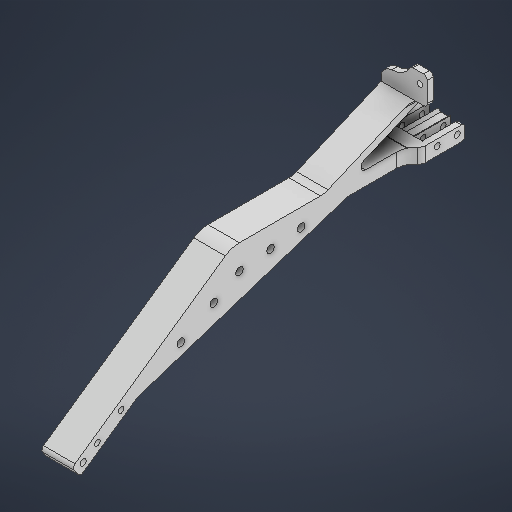
# Autodesk Inventor part: палка
Saved by Autodesk Inventor 2025 (Build 290162000, 162)
## iProperties
Created: 2025-01-21
Part Number: палка
Material: Типовые
Document SubType Name: Modeling
Designer: Phantom
Density: 1 g/cm^3
Appearance: По умолчанию
Author: Phantom
Autodesk Inventor part; units mm, degrees
ref_plane "YZ Plane" through (0, 0, 0) normal (1, 0, 0) x (0, 1, 0)
ref_plane "XZ Plane" through (0, 0, 0) normal (0, 1, 0) x (-1, 0, 0)
ref_plane "XY Plane" through (0, 0, 0) normal (0, 0, 1) x (1, 0, 0)
sketch "Эскиз1" plane through (0, 0, 0) normal (0, 0, 1) x (1, 0, 0)
  line L0 (6.1329, 20.7465) -> (8.1329, 22.2465)
  line L1 (8.1329, 22.2465) -> (8.1329, 14.2465)
  line L2 (8.1329, 14.2465) -> (6.1329, 15.7465)
  line L3 (6.1329, 15.7465) -> (2.1329, 15.7465)
  line L4 (2.1329, 15.7465) -> (0.1329, 14.2465)
  line L5 (0.1329, 14.2465) -> (0.1329, 22.2465)
  line L6 (0.1329, 22.2465) -> (2.1329, 20.7465)
  line L7 (6.1329, 20.7465) -> (2.1329, 20.7465)
  point P0 (0, 0)
  constraints: 16 end point
extrude "Выдавливание1" add sketch "Эскиз1" along normal blind 20
sketch "Эскиз2" plane through (8.1329, 14.2465, 0) normal (1, 0, 0) x (0, 0, -1)
  line L0 (-20, 0) -> (-20, 1.5) projected
  line L1 (-20, 6.5) -> (-20, 8) projected
  line L2 (-20, 8) -> (-20, 0)
  line L3 (-172, -60) -> (-160, -60) construction
  line L4 (-172, -37) -> (-205, -60)
  line L5 (-172, -37) -> (-20, 0)
  line L6 (-20, 8) -> (-175.1358, -29.7633)
  line L7 (-209.42, -53.6583) -> (-175.1358, -29.7633)
  line L8 (-205, -60) -> (-209.42, -53.6583)
  point P0 (0, -14.2465)
  constraints: 14 end point, 2 parallel, 1 horizontal, 1 perpendicular, 1 other
extrude "Выдавливание2" add sketch "Эскиз2" against normal up to surface (8 mm away)
sketch "Эскиз3" plane through (8.1329, 22.2465, 20) normal (0, 0, -1) x (-1, 0, 0)
  line L0 (0, 0) -> (2, -1.5) projected
  line L1 (2, -1.5) -> (6, -1.5) projected
  line L2 (6, -1.5) -> (8, 0) projected
  line L3 (0, 0) -> (8, 0) projected
  point P0 (8.1329, -22.2465)
extrude "Выдавливание3" cut sketch "Эскиз3" against normal blind 10
sketch "Эскиз4" plane through (0, 0, 0) normal (0, 0, -1) x (-1, 0, 0)
  line L0 (-2.1329, 20.7465) -> (-0.1329, 22.2465) projected
  line L1 (-6.1329, 20.7465) -> (-2.1329, 20.7465) projected
  line L2 (-8.1329, 22.2465) -> (-6.1329, 20.7465) projected
  line L3 (-8.1329, 14.2465) -> (-8.1329, 22.2465) projected
  line L4 (-6.1329, 15.7465) -> (-8.1329, 14.2465) projected
  line L5 (-2.1329, 15.7465) -> (-6.1329, 15.7465) projected
  line L6 (-0.1329, 14.2465) -> (-2.1329, 15.7465) projected
  line L7 (-0.1329, 22.2465) -> (-0.1329, 14.2465) projected
  line L8 (-8.1329, 18.2465) -> (-8.1329, 14.7465)
  line L9 (-8.1329, 14.2465) -> (-8.1329, 22.2465) projected
  line L10 (-8.1329, 18.2465) -> (-8.1329, 21.7465)
  line L11 (-7.6329, 21.3715) -> (-6.1329, 20.2465)
  line L12 (-8.1329, 22.2465) -> (-6.1329, 20.7465) projected
  line L13 (-6.1329, 20.2465) -> (-2.1329, 20.2465)
  line L14 (-2.1329, 20.2465) -> (-0.6329, 21.3715)
  line L15 (-8.1329, 18.2465) -> (0, 18.2465)
  line L16 (-7.6329, 15.1215) -> (-6.1329, 16.2465)
  line L17 (-6.1329, 16.2465) -> (-2.1329, 16.2465)
  line L18 (-2.1329, 16.2465) -> (-0.6329, 15.1215)
  line L19 (-8.1329, 18.2465) -> (-7.6329, 18.2465)
  line L20 (-7.6329, 21.3715) -> (-7.6329, 15.1215)
  line L21 (-4.1329, 16.2465) -> (-4.1329, 20.2465)
  line L22 (-0.6329, 21.3715) -> (-0.6329, 15.1215)
  point P0 (0, 0)
  point P1 (-0.1329, 21.7465)
  point P2 (-0.1329, 14.7465)
  dimension "d15" = 3.5
  dimension "d16" = 3.5
  constraints: 26 end point, 5 symmetric about line, 4 midpoint, 4 point on line, 3 parallel, 1 horizontal, 1 perpendicular
  measures "d15" distance of L8.start L8.end
  measures "d16" distance of L8.start L10.end
extrude "Выдавливание4" cut sketch "Эскиз4" against normal up to surface (20 mm away) contours L0 L7 L15 L22 L14 L13 L11 L20 L3 L2 L1 | L7 L6 L5 L4 L3 L15 L20 L16 L17 L18 L22
sketch "Эскиз5" plane through (8.1329, 14.2465, 20) normal (0, 0, -1) x (-1, 0, 0)
  line L0 (-11, -14.2465) -> (13, -14.2465)
  line L1 (13, -14.2465) -> (13, 14)
  line L2 (13, 14) -> (-11, 14)
  line L3 (-11, 14) -> (-11, -14.2465)
  line L4 (0, 0) -> (8, 0) projected
  line L5 (8, 8) -> (8, 0) projected
  line L6 (6, 6.5) -> (8, 8) projected
  line L7 (2, 6.5) -> (6, 6.5) projected
  line L8 (0, 8) -> (2, 6.5) projected
  line L9 (0, 0) -> (0, 8) projected
  line L10 (2, 6) -> (0.5, 7.125) projected
  line L11 (6, 6) -> (2, 6) projected
  line L12 (7.5, 7.125) -> (6, 6) projected
  line L13 (7.5, 0.875) -> (7.5, 7.125) projected
  line L14 (6, 2) -> (7.5, 0.875) projected
  line L15 (2, 2) -> (6, 2) projected
  line L16 (0.5, 0.875) -> (2, 2) projected
  line L17 (0.5, 7.125) -> (0.5, 0.875) projected
  line L18 (0, 0.875) -> (8, 0.875)
  point P0 (8.1329, -14.2465)
  constraints: 10 end point, 2 parallel, 2 perpendicular, 2 point on line, 1 horizontal
extrude "Выдавливание5" cut sketch "Эскиз5" against normal through all contours L9 L8 L7 L6 L5 L18 L13 L12 L11 L10 L17
sketch "Эскиз8" plane through (0.1329, -15.5168, 175.1358) normal (0, 0.9716279, 0.2365147) x (1, 0, 0)
  line L0 (8, 129.5409) -> (7.5, 129.5409) projected
  line L1 (8, 157.9807) -> (8, 129.5409) projected
  line L2 (7.5, 157.9807) -> (8, 157.9807) projected
  line L3 (7.5, 157.9807) -> (7.5, 129.5409) projected
  line L4 (0.5, 129.5409) -> (0, 129.5409) projected
  line L5 (0.5, 157.9807) -> (0.5, 129.5409) projected
  line L6 (0, 157.9807) -> (0.5, 157.9807) projected
  line L7 (0, 129.5409) -> (0, 157.9807) projected
  line L8 (7.5, 129.5409) -> (61, 129.5409)
  line L9 (61, 129.5409) -> (61, -147)
  line L10 (61, -147) -> (7.5, -147)
  line L11 (7.5, -147) -> (7.5, 129.5409)
  line L12 (0.5, 129.5409) -> (-35, 129.5409)
  line L13 (-35, 129.5409) -> (-35, -116)
  line L14 (-35, -116) -> (0.5, -116)
  line L15 (0.5, -116) -> (0.5, 129.5409)
  point P0 (-0.1329, 173.8368)
  point P1 (0, 129.5409)
  point P2 (8, 129.5409)
  constraints: 16 end point, 4 parallel, 2 horizontal, 2 perpendicular
extrude "Выдавливание7" cut sketch "Эскиз8" against normal blind 10
chamfer "Фаска1" distance 2 angle 45 1 edges at (4.1329, 14.2465, 20)
sketch "Эскиз9" plane through (0.1329, -39.4118, 209.42) normal (0, 0.8203982, 0.5717927) x (1, 0, 0)
  line L0 (0, 14.1297) -> (0, 34.0646) projected
  line L1 (0, 34.0646) -> (0.5, 34.0646) projected
  line L2 (0, 14.1297) -> (0, 34.0646) projected
  line L3 (0.5, 14.1297) -> (0, 14.1297) projected
  line L4 (0.5, 34.0646) -> (0.5, 14.1297) projected
  line L5 (8, 14.1297) -> (7.5, 14.1297) projected
  line L6 (8, 34.0646) -> (8, 14.1297) projected
  line L7 (7.5, 34.0646) -> (8, 34.0646) projected
  line L8 (7.5, 14.1297) -> (7.5, 34.0646) projected
  line L9 (0.5, 14.1297) -> (-8, 14.1297)
  line L10 (-8, 14.1297) -> (-8, -12)
  line L11 (-8, -12) -> (0.5, -12)
  line L12 (0.5, -12) -> (0.5, 14.1297)
  line L13 (7.5, 14.1297) -> (11, 14.1297)
  line L14 (11, 14.1297) -> (11, -15)
  line L15 (11, -15) -> (7.5, -15)
  line L16 (7.5, -15) -> (7.5, 14.1297)
  point P0 (-0.1329, 194.3431)
  point P1 (0, 34.0646)
  constraints: 16 end point, 4 parallel, 2 horizontal, 2 perpendicular
extrude "Выдавливание8" cut sketch "Эскиз9" against normal through all
sketch "Эскиз10" plane through (0.6329, 15.1215, 0) normal (-1, 0, 0) x (0, 0, 1)
  circle A0 centre (15.2, 3.125) radius 1.6
  circle A1 centre (4.2, 3.125) radius 1.6
  line L0 (0, 6.25) -> (0, 0) projected
  line L1 (15.2, 3.125) -> (0, 3.125)
  point P0 (0, -15.1215)
  constraints: 2 centre point, 2 end point, 1 midpoint
extrude "Выдавливание9" cut sketch "Эскиз10" against normal through all
sketch "Эскиз11" plane through (0.6329, 15.1215, 0) normal (-1, 0, 0) x (0, 0, 1)
  circle A0 centre (182.5992, -40.5488) radius 1.575
  arc A1 (197.0381, -49.974) -> (196.4376, -50.8354) centre (195.5197, -49.5556) ccw
  arc A2 (204.9267, -55.4731) -> (201.6465, -55.5591) centre (203.272, -54.9596) ccw
  arc A3 (201.6174, -54.4462) -> (204.8975, -54.3601) centre (203.272, -54.9596) ccw
  line L0 (209.42, -54.5333) -> (205, -60.875) projected
  circle A4 centre (195.5197, -49.5556) radius 1.575
  point P0 (0, -15.1215)
  point P1 (203.272, -54.9596)
  point P2 (203.272, -54.9596)
  point P3 (201.6465, -55.5591)
  point P4 (204.9267, -55.4731)
  dimension "d67" = 3.15
  dimension "d68" = 1.575
  constraints: 6 point on circle, 5 centre point, 1 coincident, 1 concentric
  measures "d67" diameter of A0
  measures "d68" radius of A1
extrude "Выдавливание10" cut sketch "Эскиз11" against normal through all
fillet "Сопряжение2" radius 2 2 edges at (4.1329, -45.7535, 205) (4.1329, -39.4118, 209.42)
sketch "Эскиз12" plane through (7.6329, 15.1215, 0) normal (1, 0, 0) x (0, 0, -1)
  circle A0 centre (-195.5197, -49.5556) radius 1.575 projected
  circle A1 centre (-182.5992, -40.5488) radius 1.575 projected
  circle A2 centre (-203.272, -54.9596) radius 1.7325 projected
  circle A3 centre (-4.2, 3.125) radius 1.6 projected
  circle A4 centre (-15.2, 3.125) radius 1.6 projected
  arc A5 (-207.7792, -53.3897) -> (-208.2764, -56.1741) centre (-206.6356, -55.0305) ccw projected
  line L0 (-206.1436, -59.2342) -> (-208.2764, -56.1741) projected
  arc A6 (-206.1436, -59.2342) -> (-203.3592, -59.7314) centre (-204.5028, -58.0906) ccw projected
  line L1 (-172, -37.875) -> (-203.3592, -59.7314) projected
  line L2 (-21.9433, -1.348) -> (-172, -37.875) projected
  line L3 (-20.884, 0) -> (-21.9433, -1.348) projected
  line L4 (0, 0) -> (-20.884, 0) projected
  line L5 (0, 6.25) -> (0, 0) projected
  line L6 (0, 6.25) -> (-23.5946, 6.25) projected
  line L7 (-175.1358, -30.6383) -> (-23.5946, 6.25) projected
  line L8 (-207.7792, -53.3897) -> (-175.1358, -30.6383) projected
  line L9 (-175.1358, -30.6383) -> (-122.2091, 6.25)
  line L10 (-207.7792, -53.3897) -> (-175.1358, -30.6383) projected
  line L11 (-172, -37.875) -> (-117.6576, 0)
  line L12 (-23.5946, 6.25) -> (-122.2091, 6.25)
  line L13 (-20.884, 0) -> (-117.6576, 0)
  point P0 (0, -15.1215)
  point P1 (-154.3613, -25.5814)
  point P2 (-49.2703, 0)
  constraints: 8 end point, 1 collinear, 1 horizontal, 1 parallel
extrude "Выдавливание11" add sketch "Эскиз12" against normal up to surface (7 mm away) contours L9 L12 L7 L13 L11
sketch "Эскиз13" plane through (7.6329, 15.1215, 0) normal (1, 0, 0) x (0, 0, -1)
  line L0 (-122.2091, 6.25) -> (-207.7792, -53.3897) projected
  arc A0 (-207.7792, -53.3897) -> (-208.2764, -56.1741) centre (-206.6356, -55.0305) ccw projected
  line L1 (-206.1436, -59.2342) -> (-208.2764, -56.1741) projected
  arc A1 (-206.1436, -59.2342) -> (-203.3592, -59.7314) centre (-204.5028, -58.0906) ccw projected
  line L2 (-172, -37.875) -> (-203.3592, -59.7314) projected
  line L3 (-21.9433, -1.348) -> (-172, -37.875) projected
  line L4 (-20.884, 0) -> (-21.9433, -1.348) projected
  line L5 (0, 0) -> (-20.884, 0) projected
  line L6 (0, 6.25) -> (0, 0) projected
  line L7 (0, 6.25) -> (-23.5946, 6.25) projected
  line L8 (-23.5946, 6.25) -> (-122.2091, 6.25) projected
  circle A2 centre (-195.5197, -49.5556) radius 1.575 projected
  circle A3 centre (-182.5992, -40.5488) radius 1.575 projected
  circle A4 centre (-203.272, -54.9596) radius 1.7325 projected
  circle A5 centre (-4.2, 3.125) radius 1.6 projected
  circle A6 centre (-15.2, 3.125) radius 1.6 projected
  line L9 (-154.3613, -25.5814) -> (-117.6576, 0) projected
  line L10 (-117.6576, 0) -> (-49.2703, 0) projected
  line L11 (-154.3613, -25.5814) -> (-49.2703, 0) projected
  line L12 (-154.3613, -25.5814) -> (-172, -37.875)
  line L13 (-49.2703, 0) -> (-20.884, 0)
  point P0 (0, -15.1215)
  constraints: 4 end point, 1 collinear
extrude "Выдавливание12" cut sketch "Эскиз13" against normal blind 10 contours L4 L3 L12 L11 L13
fillet "Сопряжение3" radius 13.5 2 edges at (4.1329, 21.3715, 122.2091) (4.1329, 15.1215, 117.6576)
sketch "Эскиз14" plane through (7.6329, 15.1215, 0) normal (1, 0, 0) x (0, 0, -1)
  line L0 (-203.3592, -59.7314) -> (-121.1364, -2.4246) projected
  line L1 (-187.7019, -39.3965) -> (-48.0259, 6.25)
  line L2 (-20.884, 0) -> (-113.4172, 0) projected
  line L3 (-173.6161, -39.0014) -> (-48.7504, 1.8051)
  circle A0 centre (-195.5197, -49.5556) radius 1.575 projected
  circle A1 centre (-182.5992, -40.5488) radius 1.575 projected
  circle A2 centre (-203.272, -54.9596) radius 1.7325 projected
  circle A3 centre (-4.2, 3.125) radius 1.6 projected
  circle A4 centre (-15.2, 3.125) radius 1.6 projected
  arc A5 (-117.9687, 6.25) -> (-125.6879, 3.8254) centre (-117.9687, -7.25) ccw projected
  line L4 (-125.6879, 3.8254) -> (-207.7792, -53.3897) projected
  arc A6 (-207.7792, -53.3897) -> (-208.2764, -56.1741) centre (-206.6356, -55.0305) ccw projected
  line L5 (-206.1436, -59.2342) -> (-208.2764, -56.1741) projected
  arc A7 (-206.1436, -59.2342) -> (-203.3592, -59.7314) centre (-204.5028, -58.0906) ccw projected
  line L6 (-121.1364, -2.4246) -> (-203.3592, -59.7314) projected
  arc A8 (-113.4172, 0) -> (-121.1364, -2.4246) centre (-113.4172, -13.5) ccw projected
  line L7 (-113.4172, 0) -> (-20.884, 0) projected
  line L8 (0, 0) -> (-20.884, 0) projected
  line L9 (0, 6.25) -> (0, 0) projected
  line L10 (0, 6.25) -> (-23.5946, 6.25) projected
  line L11 (-23.5946, 6.25) -> (-117.9687, 6.25) projected
  point P0 (0, -15.1215)
  point P1 (-54.2738, 0)
  point P2 (-67.1506, 0)
  point P3 (-162.2478, -31.078)
  dimension "d43" = 4
  constraints: 4 end point, 3 point on line, 1 parallel
  measures "d43" distance between parallel lines of L1 L3
extrude "Выдавливание13" add sketch "Эскиз14" against normal up to surface (7 mm away) contours L0 L1 L2 L3
sketch "Эскиз15" plane through (7.6329, 15.1215, 0) normal (1, 0, 0) x (0, 0, -1)
  line L0 (-154, -1.48) -> (-33, -1.48)
  line L1 (-113.4172, 0) -> (-67.1506, 0) projected
  line L2 (-23.5946, 6.25) -> (-117.9687, 6.25) projected
  line L3 (-33, -1.48) -> (-20.884, -1.48)
  line L4 (-20.884, -1.48) -> (-23.5946, 6.25)
  line L5 (-54.2738, 0) -> (-20.884, 0) projected
  line L6 (0, 0) -> (-20.884, 0) projected
  line L7 (0, 6.25) -> (0, 0) projected
  line L8 (0, 6.25) -> (-23.5946, 6.25) projected
  line L9 (-23.5946, 6.25) -> (-117.9687, 6.25) projected
  arc A0 (-117.9687, 6.25) -> (-125.6879, 3.8254) centre (-117.9687, -7.25) ccw projected
  line L10 (-125.6879, 3.8254) -> (-207.7792, -53.3897) projected
  arc A1 (-207.7792, -53.3897) -> (-208.2764, -56.1741) centre (-206.6356, -55.0305) ccw projected
  line L11 (-206.1436, -59.2342) -> (-208.2764, -56.1741) projected
  arc A2 (-206.1436, -59.2342) -> (-203.3592, -59.7314) centre (-204.5028, -58.0906) ccw projected
  line L12 (-173.6161, -39.0014) -> (-203.3592, -59.7314) projected
  line L13 (-173.6161, -39.0014) -> (-54.2738, 0) projected
  circle A3 centre (-195.5197, -49.5556) radius 1.575 projected
  circle A4 centre (-182.5992, -40.5488) radius 1.575 projected
  circle A5 centre (-203.272, -54.9596) radius 1.7325 projected
  circle A6 centre (-4.2, 3.125) radius 1.6 projected
  circle A7 centre (-15.2, 3.125) radius 1.6 projected
  line L14 (-67.1506, 0) -> (-162.2478, -31.078) projected
  line L15 (-121.1364, -2.4246) -> (-162.2478, -31.078) projected
  arc A8 (-113.4172, 0) -> (-121.1364, -2.4246) centre (-113.4172, -13.5) ccw projected
  line L16 (-113.4172, 0) -> (-67.1506, 0) projected
  point P0 (0, -15.1215)
  point P1 (-21.403, 0)
  point P2 (-58.8025, -1.48)
  point P3 (-119.5629, -1.48)
  point P4 (-71.6793, -1.48)
  constraints: 6 end point, 1 horizontal, 1 parallel
extrude "Выдавливание14" add sketch "Эскиз15" against normal up to surface (7 mm away) contours A8 L1 L14 L0 | L13 L5 L4 L3 L0
fillet "Сопряжение4" radius 13.5 1 edges at (4.1329, 13.6415, 20.884)
fillet "Сопряжение5" radius 2 4 edges at (4.1329, 13.6415, 58.8025) (4.1329, -23.8799, 173.6161) (4.1329, 13.6415, 71.6793) (4.1329, -15.9565, 162.2478)
sketch "Эскиз16" plane through (7.6329, 15.1215, 0) normal (1, 0, 0) x (0, 0, -1)
  arc A0 (-27.5487, -1.48) -> (-21.403, 0) centre (-27.5487, 12.02) ccw projected
  line L0 (-21.403, 0) -> (-20.884, 0) projected
  line L1 (0, 0) -> (-20.884, 0) projected
  line L2 (0, 6.25) -> (0, 0) projected
  line L3 (0, 6.25) -> (-23.5946, 6.25) projected
  line L4 (-23.5946, 6.25) -> (-117.9687, 6.25) projected
  arc A1 (-117.9687, 6.25) -> (-125.6879, 3.8254) centre (-117.9687, -7.25) ccw projected
  line L5 (-125.6879, 3.8254) -> (-207.7792, -53.3897) projected
  arc A2 (-207.7792, -53.3897) -> (-208.2764, -56.1741) centre (-206.6356, -55.0305) ccw projected
  line L6 (-206.1436, -59.2342) -> (-208.2764, -56.1741) projected
  arc A3 (-206.1436, -59.2342) -> (-203.3592, -59.7314) centre (-204.5028, -58.0906) ccw projected
  line L7 (-173.8581, -39.17) -> (-203.3592, -59.7314) projected
  arc A4 (-173.3358, -38.9098) -> (-173.8581, -39.17) centre (-172.7145, -40.8108) ccw projected
  line L8 (-173.3358, -38.9098) -> (-59.1053, -1.5789) projected
  arc A5 (-58.484, -1.48) -> (-59.1053, -1.5789) centre (-58.484, -3.48) ccw projected
  line L9 (-58.484, -1.48) -> (-27.5487, -1.48) projected
  circle A6 centre (-195.5197, -49.5556) radius 1.575 projected
  circle A7 centre (-182.5992, -40.5488) radius 1.575 projected
  circle A8 centre (-203.272, -54.9596) radius 1.7325 projected
  circle A9 centre (-4.2, 3.125) radius 1.6 projected
  circle A10 centre (-15.2, 3.125) radius 1.6 projected
  line L10 (-83.6164, -5.3811) -> (-149.3566, -26.8651) projected
  arc A11 (-151.1214, -23.3233) -> (-149.3566, -26.8651) centre (-149.9779, -24.9641) ccw projected
  line L11 (-121.1364, -2.4246) -> (-151.1214, -23.3233) projected
  arc A12 (-119.5629, -1.48) -> (-121.1364, -2.4246) centre (-113.4172, -13.5) ccw projected
  line L12 (-119.5629, -1.48) -> (-84.2377, -1.48) projected
  arc A13 (-83.6164, -5.3811) -> (-84.2377, -1.48) centre (-84.2377, -3.48) ccw projected
  line L13 (-20.884, 0) -> (-20.884, 6.25)
  point P0 (0, -15.1215)
  constraints: 2 end point, 1 perpendicular, 1 point on line
extrude "Выдавливание15" add sketch "Эскиз16" along normal blind 2.5 contours L9 A5 L8 A4 L7 A3 L6 A2 L5 A1 L4 L3 L13 L0 A0
sketch "Эскиз17" plane through (0.6329, 15.1215, 0) normal (-1, 0, 0) x (0, 0, 1)
  circle A0 centre (15.2, 3.125) radius 1.6 projected
  circle A1 centre (4.2, 3.125) radius 1.6 projected
  circle A2 centre (203.272, -54.9596) radius 1.7325 projected
  circle A3 centre (182.5992, -40.5488) radius 1.575 projected
  circle A4 centre (195.5197, -49.5556) radius 1.575 projected
  arc A5 (21.403, 0) -> (27.5487, -1.48) centre (27.5487, 12.02) ccw projected
  line L0 (27.5487, -1.48) -> (58.484, -1.48) projected
  arc A6 (59.1053, -1.5789) -> (58.484, -1.48) centre (58.484, -3.48) ccw projected
  line L1 (59.1053, -1.5789) -> (173.3358, -38.9098) projected
  arc A7 (173.8581, -39.17) -> (173.3358, -38.9098) centre (172.7145, -40.8108) ccw projected
  line L2 (203.3592, -59.7314) -> (173.8581, -39.17) projected
  arc A8 (203.3592, -59.7314) -> (206.1436, -59.2342) centre (204.5028, -58.0906) ccw projected
  line L3 (208.2764, -56.1741) -> (206.1436, -59.2342) projected
  arc A9 (208.2764, -56.1741) -> (207.7792, -53.3897) centre (206.6356, -55.0305) ccw projected
  line L4 (125.6879, 3.8254) -> (207.7792, -53.3897) projected
  arc A10 (125.6879, 3.8254) -> (117.9687, 6.25) centre (117.9687, -7.25) ccw projected
  line L5 (117.9687, 6.25) -> (23.5946, 6.25) projected
  line L6 (0, 6.25) -> (23.5946, 6.25) projected
  line L7 (0, 0) -> (0, 6.25) projected
  line L8 (20.884, 0) -> (0, 0) projected
  line L9 (20.884, 0) -> (21.403, 0) projected
  line L10 (84.2377, -1.48) -> (119.5629, -1.48) projected
  arc A11 (121.1364, -2.4246) -> (119.5629, -1.48) centre (113.4172, -13.5) ccw projected
  line L11 (151.1214, -23.3233) -> (121.1364, -2.4246) projected
  arc A12 (149.3566, -26.8651) -> (151.1214, -23.3233) centre (149.9779, -24.9641) ccw projected
  line L12 (149.3566, -26.8651) -> (83.6164, -5.3811) projected
  arc A13 (84.2377, -1.48) -> (83.6164, -5.3811) centre (84.2377, -3.48) ccw projected
  line L13 (20.884, 0) -> (20.884, 6.25) projected
  point P0 (0, -15.1215)
extrude "Выдавливание16" add sketch "Эскиз17" along normal blind 2.5 contours L9 L13 L6 L5 A10 L4 A9 L3 A8 L2 A7 L1 A6 L0 A5
sketch "Эскиз18" plane through (10.1329, 15.1215, 0) normal (1, 0, 0) x (0, 0, -1)
  line L0 (-20.2, 40.5392) -> (-20.2, 28.125) projected
  line L1 (-20.2, 28.125) -> (-20.2, 8.125) projected
  line L2 (-117.9687, 6.25) -> (-20.884, 6.25) projected
  line L3 (-71.5914, 6.25) -> (-23.4, 26.7629)
  line L4 (-61.3782, 6.25) -> (-20.2, 23.7777)
  line L5 (-20.2, 28.125) -> (-20.2, 35)
  line L6 (-20.2, 35) -> (-23.4, 35)
  line L7 (-23.4, 35) -> (-23.4, 26.7629)
  point P0 (0, -15.1215)
  point P1 (-25.2141, 6.25)
  point P2 (-30.6563, 19.3269)
  dimension "d56" = 4
  dimension "d57" = 3.2
  constraints: 10 end point, 5 point on line, 2 perpendicular, 1 parallel
  measures "d56" distance from line of L3 point (-30.656, 19.327)
  measures "d57" distance of L5.end L6.end
extrude "Выдавливание17" add sketch "Эскиз18" against normal up to surface (12 mm away)
sketch "Эскиз19" plane through (10.1329, 41.8844, 23.4) normal (0, 0, 1) x (1, 0, 0)
  line L0 (-12, 8.2371) -> (-12, 0) projected
  line L1 (0, 0) -> (-12, 0) projected
  line L2 (0, 8.2371) -> (0, 0) projected
  line L3 (0, 8.2371) -> (-12, 8.2371) projected
  line L4 (0, 0) -> (8, 0)
  line L5 (8, 0) -> (8, 15)
  line L6 (8, 15) -> (0, 15)
  line L7 (0, 15) -> (0, 0)
  line L8 (0, 8.2371) -> (-12, 8.2371) projected
  line L9 (0, 15) -> (-1, 15)
  line L10 (-1, 15) -> (-1, 8.2371)
  line L11 (-1, 8.2371) -> (0, 8.2371)
  line L12 (0, 8.2371) -> (0, 15)
  point P0 (-10.1329, -41.8844)
  point P1 (-1, 8.2371)
  constraints: 16 end point, 4 parallel, 2 horizontal, 2 perpendicular, 1 point on line
extrude "Выдавливание18" add sketch "Эскиз19" against normal up to surface (3.2 mm away) contours L10 L9 L7 L3 | L2 L7 L6 L5 L4
fillet "Сопряжение7" radius 11.75 1 edges at (9.1329, 50.1215, 21.8)
fillet "Сопряжение8" radius 2 4 edges at (9.1329, 56.8844, 21.8) (18.1329, 56.8844, 21.8) (18.1329, 41.8844, 21.8) (10.1329, 41.8844, 21.8)
sketch "Эскиз20" plane through (-1.8671, 41.8844, 23.4) normal (0, 0, 1) x (1, 0, 0)
  circle A0 centre (15.95, 9.1891) radius 1.55 projected
  point P0 (1.8671, -41.8844)
extrude "Выдавливание19" cut sketch "Эскиз20" against normal blind 10
sketch "Эскиз21" plane through (-1.8671, 15.1215, 0) normal (-1, 0, 0) x (0, 0, 1)
  circle A0 centre (203.272, -54.9596) radius 1.7325 projected
  circle A1 centre (182.5992, -40.5488) radius 1.575 projected
  circle A2 centre (195.5197, -49.5556) radius 1.575 projected
  line L0 (149.3566, -26.8651) -> (83.6164, -5.3811) projected
  arc A3 (84.2377, -1.48) -> (83.6164, -5.3811) centre (84.2377, -3.48) ccw projected
  line L1 (84.2377, -1.48) -> (119.5629, -1.48) projected
  arc A4 (121.1364, -2.4246) -> (119.5629, -1.48) centre (113.4172, -13.5) ccw projected
  line L2 (121.1364, -2.4246) -> (151.1214, -23.3233) projected
  arc A5 (149.3566, -26.8651) -> (151.1214, -23.3233) centre (149.9779, -24.9641) ccw projected
  arc A6 (21.403, 0) -> (27.5487, -1.48) centre (27.5487, 12.02) ccw projected
  line L3 (27.5487, -1.48) -> (58.484, -1.48) projected
  arc A7 (59.1053, -1.5789) -> (58.484, -1.48) centre (58.484, -3.48) ccw projected
  line L4 (59.1053, -1.5789) -> (173.3358, -38.9098) projected
  arc A8 (173.8581, -39.17) -> (173.3358, -38.9098) centre (172.7145, -40.8108) ccw projected
  line L5 (173.8581, -39.17) -> (203.3592, -59.7314) projected
  arc A9 (203.3592, -59.7314) -> (206.1436, -59.2342) centre (204.5028, -58.0906) ccw projected
  line L6 (206.1436, -59.2342) -> (208.2764, -56.1741) projected
  arc A10 (208.2764, -56.1741) -> (207.7792, -53.3897) centre (206.6356, -55.0305) ccw projected
  line L7 (207.7792, -53.3897) -> (125.6879, 3.8254) projected
  arc A11 (125.6879, 3.8254) -> (117.9687, 6.25) centre (117.9687, -7.25) ccw projected
  line L8 (117.9687, 6.25) -> (71.5914, 6.25) projected
  line L9 (23.4, 26.7629) -> (71.5914, 6.25) projected
  line L10 (23.4, 35) -> (23.4, 26.7629) projected
  line L11 (20.2, 35) -> (23.4, 35) projected
  line L12 (20.2, 23.7777) -> (20.2, 35) projected
  line L13 (61.3782, 6.25) -> (20.2, 23.7777) projected
  line L14 (61.3782, 6.25) -> (20.884, 6.25) projected
  circle A12 centre (117.9687, -7.25) radius 2.075
  circle A13 centre (84.2377, -3.48) radius 2.075
  arc A14 (149.3566, -26.8651) -> (151.1214, -23.3233) centre (149.9779, -24.9641) ccw projected
  circle A15 centre (149.9779, -24.9641) radius 2.075
  circle A16 centre (132, -15.1215) radius 2.075
  circle A17 centre (101, -5.175) radius 2.075
  line L15 (20.884, 6.25) -> (20.884, 0) projected
  line L16 (20.884, 0) -> (21.403, 0) projected
  point P0 (0, -15.1215)
  point P1 (84.7905, -1.48)
  point P2 (84.1419, -5.5528)
  point P3 (148.8311, -26.6934)
  point P4 (150.6679, -23.0072)
  dimension "d69" = 4.15
  dimension "d70" = 4.15
  dimension "d71" = 4.15
  dimension "d72" = 4.15
  dimension "d73" = 4.15
  constraints: 5 centre point, 3 coincident
  measures "d69" diameter of A12
  measures "d70" diameter of A13
  measures "d71" diameter of A15
  measures "d72" diameter of A16
  measures "d73" diameter of A17
extrude "Выдавливание20" add sketch "Эскиз21" against normal up to surface (12 mm away) contours L0 A13 L1 A4 L2 A15
sketch "Эскиз22" plane through (-1.8671, 15.1215, 0) normal (-1, 0, 0) x (0, 0, 1)
  arc A0 (84.1419, -5.5528) -> (84.7905, -1.48) centre (84.2377, -3.48) ccw projected
  circle A1 centre (84.2377, -3.48) radius 2.075
  arc A2 (150.6679, -23.0072) -> (148.8311, -26.6934) centre (149.9779, -24.9641) ccw projected
  circle A3 centre (149.9779, -24.9641) radius 2.075
  line L0 (84.1419, -5.5528) -> (83.6164, -5.3811) projected
  line L1 (150.6679, -23.0072) -> (151.1214, -23.3233) projected
  arc A4 (149.3566, -26.8651) -> (151.1214, -23.3233) centre (149.9779, -24.9641) ccw projected
  line L2 (149.3566, -26.8651) -> (148.8311, -26.6934) projected
  arc A5 (150.6679, -23.0072) -> (148.8311, -26.6934) centre (149.9779, -24.9641) ccw projected
  circle A6 centre (117.9687, -7.25) radius 2.075 projected
  circle A7 centre (132, -15.1215) radius 2.075 projected
  circle A8 centre (101, -5.175) radius 2.075 projected
  circle A9 centre (203.272, -54.9596) radius 1.7325 projected
  circle A10 centre (182.5992, -40.5488) radius 1.575 projected
  circle A11 centre (195.5197, -49.5556) radius 1.575 projected
  arc A12 (84.1419, -5.5528) -> (84.7905, -1.48) centre (84.2377, -3.48) ccw projected
  line L3 (84.1419, -5.5528) -> (83.6164, -5.3811) projected
  arc A13 (84.2377, -1.48) -> (83.6164, -5.3811) centre (84.2377, -3.48) ccw projected
  line L4 (84.2377, -1.48) -> (84.7905, -1.48) projected
  arc A14 (21.403, 0) -> (27.5487, -1.48) centre (27.5487, 12.02) ccw projected
  line L5 (27.5487, -1.48) -> (58.484, -1.48) projected
  arc A15 (59.1053, -1.5789) -> (58.484, -1.48) centre (58.484, -3.48) ccw projected
  line L6 (59.1053, -1.5789) -> (173.3358, -38.9098) projected
  arc A16 (173.8581, -39.17) -> (173.3358, -38.9098) centre (172.7145, -40.8108) ccw projected
  line L7 (173.8581, -39.17) -> (203.3592, -59.7314) projected
  arc A17 (203.3592, -59.7314) -> (206.1436, -59.2342) centre (204.5028, -58.0906) ccw projected
  line L8 (206.1436, -59.2342) -> (208.2764, -56.1741) projected
  arc A18 (208.2764, -56.1741) -> (207.7792, -53.3897) centre (206.6356, -55.0305) ccw projected
  line L9 (207.7792, -53.3897) -> (125.6879, 3.8254) projected
  arc A19 (125.6879, 3.8254) -> (117.9687, 6.25) centre (117.9687, -7.25) ccw projected
  line L10 (117.9687, 6.25) -> (71.5914, 6.25) projected
  line L11 (23.4, 26.7629) -> (71.5914, 6.25) projected
  line L12 (23.4, 35) -> (23.4, 26.7629) projected
  line L13 (20.2, 35) -> (23.4, 35) projected
  line L14 (20.2, 23.7777) -> (20.2, 35) projected
  line L15 (61.3782, 6.25) -> (20.2, 23.7777) projected
  line L16 (61.3782, 6.25) -> (20.884, 6.25) projected
  line L17 (20.884, 6.25) -> (20.884, 0) projected
  line L18 (20.884, 0) -> (21.403, 0) projected
  point P0 (0, -15.1215)
  point P1 (148.8311, -26.6934)
  point P2 (83.6164, -5.3811)
  point P3 (84.7905, -1.48)
  point P4 (84.1419, -5.5528)
  constraints: 2 centre point, 2 coincident, 1 concentric
extrude "Выдавливание21" cut sketch "Эскиз22" against normal through all contours A1 L4 A13 L0 | L1 A4 L2 A2 | A3 L2 A4 L1
sketch "Эскиз23" plane through (10.1329, 13.6415, 27.5487) normal (0, -1, 0) x (1, 0, 0)
  line L0 (-14, -7.3487) -> (-14, -27.5487) projected
  line L1 (2, -7.3487) -> (2, -27.5487) projected
  line L2 (-14, -27.5487) -> (-17.2, -27.5487)
  line L3 (-17.2, -27.5487) -> (-17.2, -7.3487)
  line L4 (-17.2, -7.3487) -> (-14, -7.3487)
  line L5 (-14, -7.3487) -> (-14, -27.5487)
  line L6 (2, -27.5487) -> (5.2, -27.5487)
  line L7 (5.2, -27.5487) -> (5.2, -7.3487)
  line L8 (5.2, -7.3487) -> (2, -7.3487)
  line L9 (2, -7.3487) -> (2, -27.5487)
  line L10 (-12, -7.3487) -> (-12, -4.1487) projected
  line L11 (-12, -7.3487) -> (-17.2, -7.3487)
  line L12 (-17.2, -7.3487) -> (-17.2, -4.1487)
  line L13 (-17.2, -4.1487) -> (-12, -4.1487)
  line L14 (-12, -4.1487) -> (-12, -7.3487)
  line L15 (0, 33.8296) -> (0, -7.3487) projected
  line L16 (5.2, -7.3487) -> (0, -7.3487)
  line L17 (0, -7.3487) -> (0, -4.1487)
  line L18 (0, -4.1487) -> (5.2, -4.1487)
  line L19 (5.2, -4.1487) -> (5.2, -7.3487)
  line L20 (0, 0) -> (0, -6.1457) projected
  line L21 (0, 0) -> (-12, 0) projected
  line L22 (-12, -6.1457) -> (-12, 0) projected
  line L23 (0, -6.1457) -> (-12, -6.1457) projected
  line L24 (-12, -4.1487) -> (-11.6593, -4.1487)
  line L25 (0, -4.1487) -> (-0.3407, -4.1487)
  line L26 (-12, -7.3487) -> (0, -7.3487)
  point P0 (-10.1329, -27.5487)
  point P1 (-1.7635, -6.1457)
  dimension "d78" = 3.2
  dimension "d79" = 3.2
  constraints: 38 end point, 8 parallel, 6 horizontal, 5 point on line, 4 perpendicular, 1 other
  measures "d78" distance of L3.end L4.end
  measures "d79" distance of L8.end L7.end
extrude "Выдавливание22" add sketch "Эскиз23" against normal blind 8
fillet "Сопряжение9" radius 10.25 6 edges at (10.1329, 17.8332, 23.3999) (10.1329, 13.9682, 23.3999) (10.1329, 21.5065, 23.3999) (-1.8671, 17.8332, 23.3999) (-1.8671, 13.9682, 23.3999) (-1.8671, 21.5065, 23.3999)
fillet "Сопряжение10" radius 3.75 6 edges at (-7.0671, 13.9682, 23.3999) (-7.0671, 17.8332, 23.3999) (-7.0671, 21.5065, 23.3999) (15.3329, 13.9682, 23.3999) (15.3329, 17.8332, 23.3999) (15.3329, 21.5065, 23.3999)
sketch "Эскиз24" plane through (15.3329, 13.6415, 0) normal (1, 0, 0) x (0, 0, -1)
  circle A0 centre (-15.2, 4.605) radius 1.6 projected
  circle A1 centre (-4.2, 4.605) radius 1.6 projected
  point P0 (0, -13.6415)
extrude "Выдавливание23" cut sketch "Эскиз24" against normal through all
fillet "Сопряжение11" radius 2 4 edges at (13.7329, 13.6415, 0) (13.7329, 21.6415, 0) (-5.4671, 13.6415, 0) (-5.4671, 21.6415, 0)
fillet "Сопряжение13" radius 10.5 1 edges at (4.1329, 21.3715, 71.5914)
fillet "Сопряжение14" radius 2.5 1 edges at (4.1329, 21.3715, 61.3782)
sketch "Эскиз25" plane through (-1.8671, 15.1215, 0) normal (-1, 0, 0) x (0, 0, 1)
  circle A0 centre (203.272, -54.9596) radius 1.7325 projected
  circle A1 centre (182.5992, -40.5488) radius 1.575 projected
  circle A2 centre (195.5197, -49.5556) radius 1.575 projected
  circle A3 centre (84.2377, -3.48) radius 2.075 projected
  circle A4 centre (101, -5.175) radius 2.075 projected
  circle A5 centre (132, -15.1215) radius 2.075 projected
  circle A6 centre (117.9687, -7.25) radius 2.075 projected
  circle A7 centre (149.9779, -24.9641) radius 2.075 projected
  line L0 (20.2, 23.7777) -> (20.2, 35) projected
  line L1 (50.1008, 11.0503) -> (20.2, 23.7777) projected
  arc A8 (49.1217, 6.25) -> (50.1008, 11.0503) centre (49.1217, 8.75) ccw projected
  line L2 (49.1217, 6.25) -> (32.3196, 6.25) projected
  line L3 (32.3196, -1.48) -> (32.3196, 6.25) projected
  line L4 (58.484, -1.48) -> (32.3196, -1.48) projected
  arc A9 (59.1053, -1.5789) -> (58.484, -1.48) centre (58.484, -3.48) ccw projected
  line L5 (59.1053, -1.5789) -> (173.3358, -38.9098) projected
  arc A10 (173.8581, -39.17) -> (173.3358, -38.9098) centre (172.7145, -40.8108) ccw projected
  line L6 (173.8581, -39.17) -> (203.3592, -59.7314) projected
  arc A11 (203.3592, -59.7314) -> (206.1436, -59.2342) centre (204.5028, -58.0906) ccw projected
  line L7 (206.1436, -59.2342) -> (208.2764, -56.1741) projected
  arc A12 (208.2764, -56.1741) -> (207.7792, -53.3897) centre (206.6356, -55.0305) ccw projected
  line L8 (207.7792, -53.3897) -> (125.6879, 3.8254) projected
  arc A13 (125.6879, 3.8254) -> (117.9687, 6.25) centre (117.9687, -7.25) ccw projected
  line L9 (117.9687, 6.25) -> (73.7331, 6.25) projected
  arc A14 (69.6208, 7.0888) -> (73.7331, 6.25) centre (73.7331, 16.75) ccw projected
  line L10 (23.4, 26.7629) -> (69.6208, 7.0888) projected
  line L11 (23.4, 35) -> (23.4, 26.7629) projected
  line L12 (24.3476, -1.48) -> (24.3476, 6.52) projected
  line L13 (32.3196, -1.48) -> (24.3476, -1.48) projected
  line L14 (32.3196, -1.48) -> (32.3196, 6.25) projected
  line L15 (27.5487, 6.25) -> (32.3196, 6.25) projected
  line L16 (27.5487, 6.25) -> (27.5487, 6.52) projected
  line L17 (24.3476, 6.52) -> (27.5487, 6.52) projected
  line L18 (24.3476, 6.52) -> (21.431, 6.52) projected
  line L19 (21.431, 6.52) -> (21.431, -1.48) projected
  line L20 (21.431, -1.48) -> (24.3476, -1.48) projected
  line L21 (24.3476, -1.48) -> (24.3476, 6.52) projected
  line L22 (0, 1.125) -> (20, 1.125) projected
  circle A15 centre (4.2, 3.125) radius 1.6 projected
  circle A16 centre (15.2, 3.125) radius 1.6 projected
  arc A17 (2, 6.52) -> (0, 4.52) centre (2, 4.52) ccw projected
  line L23 (0, 0.52) -> (0, 4.52) projected
  arc A18 (0, 0.52) -> (2, -1.48) centre (2, 0.52) ccw projected
  line L24 (21.431, -1.48) -> (2, -1.48) projected
  line L25 (21.431, 6.52) -> (21.431, -1.48) projected
  line L26 (2, 6.52) -> (21.431, 6.52) projected
  line L27 (23.4, 29.7407) -> (23.4, 35.6467) projected
  line L28 (23.4, 35.6467) -> (20.2, 35.6467) projected
  line L29 (20.2, 35.6467) -> (20.2, 29.7407) projected
  line L30 (20.2, 29.7407) -> (23.4, 29.7407) projected
  line L31 (23.4, 37.502) -> (20.2, 37.502) projected
  line L32 (20.2, 41.7629) -> (20.2, 40.7792) projected
  line L33 (20.2, 40.7792) -> (23.4, 40.7792) projected
  line L34 (23.4, 40.7792) -> (23.4, 41.7629) projected
  line L35 (23.4, 41.7629) -> (20.2, 41.7629) projected
  line L36 (20.2, 35) -> (23.4, 35) projected
  point P0 (0, -15.1215)
extrude "Выдавливание24" add sketch "Эскиз25" along normal up to surface (5.2 mm away) contours L0 L30 L11 L10 A14 L9 A13 L8 A12 L7 A11 L6 A10 L5 A9 L4 L3 L2 A8 L1 | L0 L36 L11 L30 | L3 L13 L12 L17 L16 L15 | L20 L19 L18 L12
fillet "Сопряжение15" radius 6 1 edges at (-7.0671, 50.1215, 21.8)
